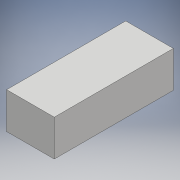
# Autodesk Inventor part: CRANEJ2
Saved by Autodesk Inventor 2017 (Build 210142000, 142)
## iProperties
Part Number: CRANEJ2
Material: 一般
Document SubType Name: Modeling
Designer: rsdlab
Density: 1 g/cm^3
Appearance: 既定
Author: rsdlab
Autodesk Inventor part; units mm, degrees
ref_plane "YZ Plane" through (0, 0, 0) normal (1, 0, 0) x (0, 1, 0)
ref_plane "XZ Plane" through (0, 0, 0) normal (0, 1, 0) x (-1, 0, 0)
ref_plane "XY Plane" through (0, 0, 0) normal (0, 0, 1) x (1, 0, 0)
sketch "スケッチ1" plane through (0, 0, 0) normal (0, 1, 0) x (-1, 0, 0)
  line L0 (0, 0) -> (0.42, 0)
  line L1 (0.42, 0) -> (0.42, -0.32)
  line L2 (0.42, -0.32) -> (0, -0.32)
  line L3 (0, -0.32) -> (0, 0)
  dimension "d0" = 0.42
  dimension "d1" = 0.32
  constraints: 8 end point, 2 parallel, 1 horizontal, 1 perpendicular
  measures "d0" distance of L1.end L2.end
  measures "d1" distance of L0.end L1.end
extrude "押し出し1" add sketch "スケッチ1" against normal blind 1.05
